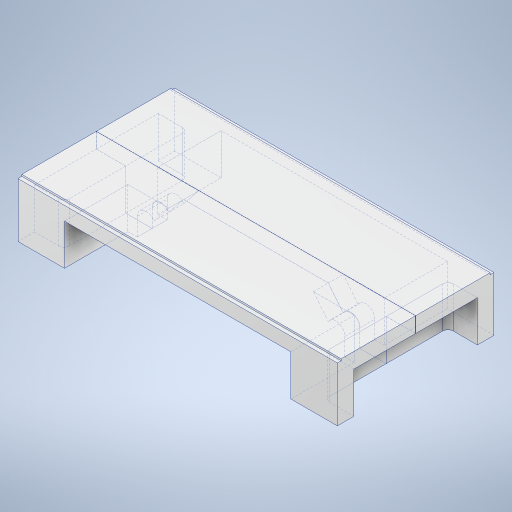
# Autodesk Inventor part: ZadBabkaOsnova
Saved by Autodesk Inventor 2024 (Build 280153000, 153)
## iProperties
Created: 2023-08-28
Part Number: ZadBabkaOsnova
Material: Aluminum 6061
Document SubType Name: Modeling
Designer: KirikDK
Density: 2.7 g/cm^3
Appearance: Aluminum - Flat
Mass: 4409.76 g
Surface Area: 2192.33 cm^2
Volume: 1633.24 cm^3
Author: KirikDK
Autodesk Inventor part; units mm, degrees
ref_plane "YZ Plane" through (0, 0, 0) normal (1, 0, 0) x (0, 1, 0)
ref_plane "XZ Plane" through (0, 0, 0) normal (0, 1, 0) x (-1, 0, 0)
ref_plane "XY Plane" through (0, 0, 0) normal (0, 0, 1) x (1, 0, 0)
sketch "Sketch1" plane through (0, 0, 0) normal (0, 1, 0) x (-1, 0, 0)
  line L0 (50, 50) -> (-125, 50)
  line L1 (-125, 50) -> (-125, -125)
  line L2 (-125, -125) -> (50, -125)
  line L3 (50, -125) -> (50, 50)
  point P0 (0, 0)
  dimension "d0" = 175
  dimension "d1" = 175
  constraints: 8 end point, 2 parallel, 1 horizontal, 1 perpendicular
  measures "d0" distance of L2.end L0.start
  measures "d1" distance of L0.start L0.end
extrude "Extrusion1" add sketch "Sketch1" along normal blind 12
sketch "Sketch2" plane through (0, 12, 0) normal (0, 1, 0) x (1, 0, 0)
  line L0 (-50, -50) -> (125, -50) projected
  line L1 (-150, -50) -> (225, -50)
  line L2 (225, -50) -> (225, 125)
  line L3 (225, 125) -> (-150, 125)
  line L4 (-150, 125) -> (-150, -50)
  line L5 (-50, 125) -> (-50, -50) projected
  line L6 (125, -50) -> (125, 125) projected
  point P0 (0, 0)
  point P1 (55, -50)
  dimension "d8" = 100
  dimension "d9" = 100
  constraints: 8 end point, 2 parallel, 1 horizontal, 1 perpendicular, 1 point on line
  measures "d8" distance between parallel lines of L6 L2
  measures "d9" distance between parallel lines of L5 L4
extrude "Extrusion2" add sketch "Sketch2" against normal blind 18
sketch "Sketch3" plane through (0, 0, 0) normal (0, -1, 0) x (1, 0, 0)
  line L0 (225, 50) -> (-150, 50) projected
  line L1 (-150, 50) -> (-150, -125) projected
  line L2 (-150, -125) -> (225, -125) projected
  line L3 (225, -125) -> (225, 50) projected
  line L4 (-115.4465, 50) -> (-95.4465, 50)
  line L5 (-95.4465, 50) -> (-95.4465, -125)
  line L6 (-95.4465, -125) -> (-115.4465, -125)
  line L7 (-115.4465, -125) -> (-115.4465, 50)
  line L8 (190.4465, 50) -> (170.4465, 50)
  line L9 (170.4465, 50) -> (170.4465, -125)
  line L10 (170.4465, -125) -> (190.4465, -125)
  line L11 (190.4465, -125) -> (190.4465, 50)
  line L12 (-150, -125) -> (-115.4465, -125)
  line L13 (-115.4465, -125) -> (-115.4465, -110)
  line L14 (-115.4465, -110) -> (-150, -110)
  line L15 (-150, -110) -> (-150, -125)
  line L16 (-150, 50) -> (-115.4465, 50)
  line L17 (-115.4465, 50) -> (-115.4465, 35)
  line L18 (-115.4465, 35) -> (-150, 35)
  line L19 (-150, 35) -> (-150, 50)
  line L20 (190.4465, 50) -> (225, 50)
  line L21 (225, 50) -> (225, 35)
  line L22 (225, 35) -> (190.4465, 35)
  line L23 (190.4465, 35) -> (190.4465, 50)
  line L24 (190.4465, -125) -> (225, -125)
  line L25 (225, -125) -> (225, -110)
  line L26 (225, -110) -> (190.4465, -110)
  line L27 (190.4465, -110) -> (190.4465, -125)
  line L28 (-95.4465, -20) -> (-45.4465, -20)
  line L29 (-45.4465, -20) -> (-45.4465, -55)
  line L30 (-45.4465, -55) -> (-95.4465, -55)
  line L31 (-95.4465, -55) -> (-95.4465, -20)
  line L32 (170.4465, -20) -> (120.4465, -20)
  line L33 (120.4465, -20) -> (120.4465, -55)
  line L34 (120.4465, -55) -> (170.4465, -55)
  line L35 (170.4465, -55) -> (170.4465, -20)
  point P0 (0, 0)
  point P1 (190.4465, -125)
  point P2 (170.4465, 50)
  dimension "d10" = 265.893
  dimension "d11" = 20
  dimension "d12" = 20
  dimension "d13" = 34.5535
  dimension "d14" = 34.5535
  dimension "d17" = 15
  dimension "d18" = 15
  dimension "d19" = 15
  dimension "d20" = 15
  dimension "d22" = 50
  dimension "d23" = 50
  dimension "d24" = 70
  dimension "d25" = 70
  constraints: 64 end point, 16 parallel, 12 point on line, 8 horizontal, 8 perpendicular
  measures "d10" distance between parallel lines of L9 L5
  measures "d11" distance between parallel lines of L5 L7
  measures "d12" distance between parallel lines of L11 L9
  measures "d13" distance between parallel lines of L3 L11
  measures "d14" distance between parallel lines of L1 L7
  measures "d17" distance between parallel lines of L2 L26
  measures "d18" distance between parallel lines of L0 L22
  measures "d19" distance between parallel lines of L12 L14
  measures "d20" distance between parallel lines of L0 L18
  measures "d22" distance between parallel lines of L35 L33
  measures "d23" distance between parallel lines of L5 L29
  measures "d24" distance between parallel lines of L0 L28
  measures "d25" distance between parallel lines of L2 L30
extrude "Extrusion3" add sketch "Sketch3" along normal blind 48 contours L3 L22 L11 L0 | L11 L2 L9 L0 | L3 L2 L11 L26 | L5 L2 L7 L0 | L9 L34 L33 L32 | L7 L18 L1 L0 | L28 L29 L30 L5 | L7 L2 L1 L14
fillet "Fillet1" radius 6 4 edges at (-115.4465, -27, -110) (-115.4465, -27, 35) (190.4465, -27, 35) (190.4465, -27, -110)
sketch "Sketch4" plane through (0, -48, 0) normal (0, -1, 0) x (1, 0, 0)
  point P0 (0, 0)
sketch "Sketch5" plane through (120.4465, -6, -20) normal (0, 0, 1) x (1, 0, 0)
  circle A0 centre (28.5535, -26.925) radius 10.5
  circle A1 centre (-194.4465, -26.925) radius 10.5
  line L0 (-215.893, 0) -> (-215.893, -42) projected
  line L1 (50, 0) -> (50, -42) projected
  line L2 (50, 0) -> (-215.893, 0) projected
  line L3 (2, 0) -> (0, 0)
  line L4 (0, 0) -> (0, -42) projected
  line L5 (0, -42) -> (12, -42)
  line L6 (12, -42) -> (28.5535, -26.925)
  line L7 (-165.893, 0) -> (-165.893, -42) projected
  line L8 (-167.893, 0) -> (-165.893, 0)
  line L9 (-165.893, -42) -> (-215.893, -42) projected
  line L10 (-165.893, 0) -> (-165.893, -42)
  line L11 (-165.893, -42) -> (-194.4465, -42)
  line L12 (-194.4465, -42) -> (-194.4465, -26.925)
  line L13 (-204.9465, -26.925) -> (-194.4465, -26.925)
  line L14 (-194.4465, -26.925) -> (-194.4465, -42)
  line L15 (-194.4465, -42) -> (-204.9465, -42)
  line L16 (-204.9465, -42) -> (-204.9465, -26.925)
  line L17 (39.0535, -26.925) -> (12, -26.925)
  line L18 (12, -26.925) -> (12, -42)
  line L19 (12, -42) -> (39.0535, -42)
  line L20 (39.0535, -42) -> (39.0535, -26.925)
  line L21 (-194.4465, -26.925) -> (-189.4465, -26.925)
  line L22 (28.5535, -26.925) -> (23.5535, -26.925)
  line L23 (23.5535, -26.925) -> (2, 0)
  line L24 (-189.4465, -26.925) -> (-167.893, 0)
  point P0 (-120.4465, 6)
  point P1 (20.7903, -33.9948)
  point P2 (-194.4465, -37.425)
  point P3 (19.4147, -21.7547)
  point P4 (2, 0)
  point P5 (-185.3077, -21.7547)
  point P6 (-167.893, 0)
  dimension "d32" = 21
  dimension "d33" = 21
  dimension "d26" = 223
  dimension "d27" = 21.4465
  dimension "d29" = 26.925
  dimension "d30" = 26.925
  dimension "d31" = 21.4465
  dimension "d34" = 12
  dimension "d35" = 2
  dimension "d37" = 2
  dimension "d40" = 5
  dimension "d41" = 5
  constraints: 38 end point, 4 parallel, 4 perpendicular, 3 horizontal, 3 point on line, 6 other
  measures "d26" distance of point (28.554, -26.925) L12.end
  measures "d27" distance from line of L0 L12.end
  measures "d29" distance from line of L2 point (28.554, -26.925)
  measures "d30" distance from line of L2 L12.end
  measures "d31" distance from line of L1 point (28.554, -26.925)
  measures "d34" distance of L4.end L5.end
  measures "d35" distance of L3.start L3.end
  measures "d37" distance of L7.start L8.start
  measures "d40" distance of L21.end L12.end
  measures "d41" distance of point (28.554, -26.925) L22.end
extrude "Extrusion4" cut sketch "Sketch5" against normal blind 54 contours L17 L23 A0 | L20 L19 L6 A0 | A0 L6 L17 | L7 L9 L12 A1 L24 L2 | L23 L17 A0 | A0 L17 L18 L5 L4 L2 L23 | L6 L18 L17 A0 | A0 L17 L6 | L24 L21 L13 A1 | A1 L12 L21 L24 | L9 L16 A1 L12 | L13 L12 A1
sketch "Sketch6" plane through (0, -48, 0) normal (0, -1, 0) x (1, 0, 0)
  line L0 (-168, -37.45) -> (251, -37.45)
  line L1 (251, -37.45) -> (251, -37.55)
  line L2 (251, -37.55) -> (-168, -37.55)
  line L3 (-168, -37.55) -> (-168, -37.45)
  line L4 (170.4465, 50) -> (-95.4465, 50) projected
  line L5 (-95.4465, -125) -> (170.4465, -125) projected
  point P0 (0, 0)
  dimension "d42" = 87.45
  dimension "d43" = 87.45
  constraints: 8 end point, 2 parallel, 1 horizontal, 1 perpendicular
  measures "d42" distance between parallel lines of L4 L0
  measures "d43" distance between parallel lines of L5 L2
extrude "Extrusion5" cut sketch "Sketch6" against normal blind 98
sketch "Sketch7" plane through (0, -48, 0) normal (0, -1, 0) x (1, 0, 0)
  line L0 (-115.4465, -37.45) -> (-84.5, -37.45) projected
  line L1 (-84.5, -37.45) -> (-84.5, -20) projected
  line L2 (-84.5, -20) -> (-95.4465, -20) projected
  line L3 (-95.4465, -20) -> (-95.4465, 50) projected
  line L4 (-95.4465, 50) -> (-150, 50) projected
  line L5 (-150, 50) -> (-150, 35) projected
  line L6 (-150, 35) -> (-121.4465, 35) projected
  arc A0 (-115.4465, 29) -> (-121.4465, 35) centre (-121.4465, 29) ccw projected
  line L7 (-115.4465, 29) -> (-115.4465, -37.45) projected
  line L8 (-84.5, -37.55) -> (-115.4465, -37.55) projected
  line L9 (-115.4465, -37.55) -> (-115.4465, -104) projected
  arc A1 (-121.4465, -110) -> (-115.4465, -104) centre (-121.4465, -104) ccw projected
  line L10 (-121.4465, -110) -> (-150, -110) projected
  line L11 (-150, -110) -> (-150, -125) projected
  line L12 (-150, -125) -> (-95.4465, -125) projected
  line L13 (-95.4465, -125) -> (-95.4465, -55) projected
  line L14 (-95.4465, -55) -> (-84.5, -55) projected
  line L15 (-84.5, -55) -> (-84.5, -37.55) projected
  line L16 (159.5, -37.45) -> (190.4465, -37.45) projected
  line L17 (190.4465, -37.45) -> (190.4465, 29) projected
  arc A2 (196.4465, 35) -> (190.4465, 29) centre (196.4465, 29) ccw projected
  line L18 (196.4465, 35) -> (225, 35) projected
  line L19 (225, 35) -> (225, 50) projected
  line L20 (225, 50) -> (170.4465, 50) projected
  line L21 (170.4465, 50) -> (170.4465, -20) projected
  line L22 (170.4465, -20) -> (159.5, -20) projected
  line L23 (159.5, -20) -> (159.5, -37.45) projected
  line L24 (190.4465, -37.55) -> (159.5, -37.55) projected
  line L25 (159.5, -37.55) -> (159.5, -55) projected
  line L26 (159.5, -55) -> (170.4465, -55) projected
  line L27 (170.4465, -55) -> (170.4465, -125) projected
  line L28 (170.4465, -125) -> (225, -125) projected
  line L29 (225, -125) -> (225, -110) projected
  line L30 (225, -110) -> (196.4465, -110) projected
  arc A3 (190.4465, -104) -> (196.4465, -110) centre (196.4465, -104) ccw projected
  line L31 (190.4465, -104) -> (190.4465, -37.55) projected
  point P0 (0, 0)
extrude "Extrusion6" add sketch "Sketch7" along normal blind 6
sketch "Sketch8" plane through (-150, 12, 50) normal (0, 0, 1) x (1, 0, 0)
  line L0 (375, 0) -> (375, -66) projected
  line L1 (0, 0) -> (375, 0) projected
  line L2 (0, 0) -> (0, -66) projected
  line L3 (54.5535, -66) -> (0, -66) projected
  line L4 (54.5535, -18) -> (54.5535, -66) projected
  line L5 (320.4465, -18) -> (54.5535, -18) projected
  line L6 (320.4465, -18) -> (320.4465, -66) projected
  line L7 (375, -66) -> (320.4465, -66) projected
  line L8 (0, 0) -> (375, 0)
  line L9 (375, 0) -> (375, -2)
  line L10 (375, -2) -> (0, -2)
  line L11 (0, -2) -> (0, 0)
  point P0 (150, -12)
  point P1 (375, -2)
  point P2 (0, -2)
  constraints: 8 end point, 2 parallel, 1 horizontal, 1 perpendicular
extrude "Extrusion7" add sketch "Sketch8" along normal blind 4.5 contours L0 L7 L6 L5 L4 L3 L2 L10
sketch "Sketch9" plane through (225, 12, -125) normal (0, 0, -1) x (-1, 0, 0)
  line L0 (320.4465, -18) -> (54.5535, -18) projected
  line L1 (320.4465, -18) -> (320.4465, -66) projected
  line L2 (375, -66) -> (320.4465, -66) projected
  line L3 (375, 0) -> (375, -66) projected
  line L4 (0, 0) -> (375, 0) projected
  line L5 (0, 0) -> (0, -66) projected
  line L6 (54.5535, -66) -> (0, -66) projected
  line L7 (54.5535, -18) -> (54.5535, -66) projected
  line L8 (375, 0) -> (0, 0)
  line L9 (0, 0) -> (0, -2)
  line L10 (0, -2) -> (375, -2)
  line L11 (375, -2) -> (375, 0)
  point P0 (225, -12)
  point P1 (375, -2)
  constraints: 8 end point, 2 parallel, 1 horizontal, 1 perpendicular, 1 point on line
extrude "Extrusion8" add sketch "Sketch9" along normal blind 4.5 contours L0 L7 L6 L5 L10 L3 L2 L1
body "Solid1"
